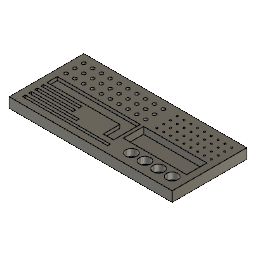
ToolingHolder1 v16 (Autodesk Fusion 360 design; units mm, degrees)
Autodesk Fusion 360 part; units mm, degrees
sketch "Sketch1" plane through (0, 0, 0) normal (0, 0, 1) x (1, 0, 0)
  line L0 (0, 0) -> (304.8, 0)
  line L1 (304.8, 0) -> (304.8, 139.7)
  line L2 (304.8, 139.7) -> (0, 139.7)
  line L3 (0, 139.7) -> (0, 0)
  dimension "d1" = 139.7
  dimension "d2" = 304.8
extrude "Extrude1" add sketch "Sketch1" along normal blind 19.05
sketch "Sketch2" plane through (0, 0, 19.05) normal (0, 0, 1) x (-1, 0, 0)
  line L0 (0, -139.7) -> (0, 0)
  line L1 (0, 0) -> (-304.8, 0)
  line L2 (-304.8, 0) -> (-304.8, -139.7)
  line L3 (-304.8, -139.7) -> (0, -139.7)
  line L4 (-304.8, -139.7) -> (0, -139.7)
  line L5 (-304.8, 0) -> (-304.8, -139.7)
  line L6 (0, 0) -> (-304.8, 0)
  line L7 (0, -139.7) -> (0, 0)
  line L8 (-12.7, -12.7) -> (-292.1, -12.7)
  line L9 (-292.1, -12.7) -> (-292.1, -127)
  line L10 (-292.1, -127) -> (-12.7, -127)
  line L11 (-12.7, -127) -> (-12.7, -12.7)
  circle A0 centre (-281.686, -23.114) radius 10.414
  circle A1 centre (-256.286, -23.114) radius 10.414
  line L12 (-12.7, -12.7) -> (-171.45, -12.7)
  line L13 (-171.45, -12.7) -> (-171.45, -17.78)
  line L14 (-171.45, -17.78) -> (-12.7, -17.78)
  line L15 (-12.7, -17.78) -> (-12.7, -12.7)
  line L16 (-12.7, -24.13) -> (-101.6, -24.13)
  line L17 (-101.6, -24.13) -> (-101.6, -29.21)
  line L18 (-101.6, -29.21) -> (-12.7, -29.21)
  line L19 (-12.7, -29.21) -> (-12.7, -24.13)
  line L20 (-12.7, -35.56) -> (-83.82, -35.56)
  line L21 (-83.82, -35.56) -> (-83.82, -40.64)
  line L22 (-83.82, -40.64) -> (-12.7, -40.64)
  line L23 (-12.7, -40.64) -> (-12.7, -35.56)
  line L24 (-12.7, -46.99) -> (-83.82, -46.99)
  line L25 (-83.82, -46.99) -> (-83.82, -52.07)
  line L26 (-83.82, -52.07) -> (-12.7, -52.07)
  line L27 (-12.7, -52.07) -> (-12.7, -46.99)
  circle A2 centre (-230.886, -23.114) radius 10.414
  circle A3 centre (-205.486, -23.114) radius 10.414
  line L28 (-12.7, -77.47) -> (-167.64, -77.47)
  line L29 (-167.64, -77.47) -> (-167.64, -27.615)
  line L30 (-167.64, -27.615) -> (-148.59, -27.615)
  line L31 (-148.59, -27.615) -> (-148.59, -58.42)
  line L32 (-148.59, -58.42) -> (-12.7, -58.42)
  circle A4 centre (-15.875, -123.825) radius 3.175
  circle A5 centre (-32.385, -123.825) radius 3.175
  circle A6 centre (-48.895, -123.825) radius 3.175
  circle A7 centre (-65.405, -123.825) radius 3.175
  circle A8 centre (-81.915, -123.825) radius 3.175
  circle A9 centre (-98.425, -123.825) radius 3.175
  circle A10 centre (-114.935, -123.825) radius 3.175
  circle A11 centre (-131.445, -123.825) radius 3.175
  circle A12 centre (-147.955, -123.825) radius 3.175
  circle A13 centre (-164.465, -123.825) radius 3.175
  circle A14 centre (-15.875, -107.315) radius 3.175
  circle A15 centre (-32.385, -107.315) radius 3.175
  circle A16 centre (-48.895, -107.315) radius 3.175
  circle A17 centre (-65.405, -107.315) radius 3.175
  circle A18 centre (-81.915, -107.315) radius 3.175
  circle A19 centre (-98.425, -107.315) radius 3.175
  circle A20 centre (-114.935, -107.315) radius 3.175
  circle A21 centre (-131.445, -107.315) radius 3.175
  circle A22 centre (-147.955, -107.315) radius 3.175
  circle A23 centre (-164.465, -107.315) radius 3.175
  circle A24 centre (-15.875, -90.805) radius 3.175
  circle A25 centre (-32.385, -90.805) radius 3.175
  circle A26 centre (-48.895, -90.805) radius 3.175
  circle A27 centre (-65.405, -90.805) radius 3.175
  circle A28 centre (-81.915, -90.805) radius 3.175
  circle A29 centre (-98.425, -90.805) radius 3.175
  circle A30 centre (-114.935, -90.805) radius 3.175
  circle A31 centre (-131.445, -90.805) radius 3.175
  circle A32 centre (-147.955, -90.805) radius 3.175
  circle A33 centre (-164.465, -90.805) radius 3.175
  circle A34 centre (-290.5125, -125.4125) radius 1.5875
  line L33 (-173.99, -77.47) -> (-292.1, -77.47)
  line L34 (-292.1, -77.47) -> (-292.1, -39.624)
  line L35 (-292.1, -39.624) -> (-173.99, -39.624)
  line L36 (-173.99, -39.624) -> (-173.99, -77.47)
  circle A35 centre (-277.8125, -125.4125) radius 1.5875
  circle A36 centre (-265.1125, -125.4125) radius 1.5875
  circle A37 centre (-252.4125, -125.4125) radius 1.5875
  circle A38 centre (-239.7125, -125.4125) radius 1.5875
  circle A39 centre (-227.0125, -125.4125) radius 1.5875
  circle A40 centre (-214.3125, -125.4125) radius 1.5875
  circle A41 centre (-201.6125, -125.4125) radius 1.5875
  circle A42 centre (-188.9125, -125.4125) radius 1.5875
  circle A43 centre (-290.5125, -112.7125) radius 1.5875
  circle A44 centre (-277.8125, -112.7125) radius 1.5875
  circle A45 centre (-265.1125, -112.7125) radius 1.5875
  circle A46 centre (-252.4125, -112.7125) radius 1.5875
  circle A47 centre (-239.7125, -112.7125) radius 1.5875
  circle A48 centre (-227.0125, -112.7125) radius 1.5875
  circle A49 centre (-214.3125, -112.7125) radius 1.5875
  circle A50 centre (-201.6125, -112.7125) radius 1.5875
  circle A51 centre (-188.9125, -112.7125) radius 1.5875
  circle A52 centre (-290.5125, -100.0125) radius 1.5875
  circle A53 centre (-277.8125, -100.0125) radius 1.5875
  circle A54 centre (-265.1125, -100.0125) radius 1.5875
  circle A55 centre (-252.4125, -100.0125) radius 1.5875
  circle A56 centre (-239.7125, -100.0125) radius 1.5875
  circle A57 centre (-227.0125, -100.0125) radius 1.5875
  circle A58 centre (-214.3125, -100.0125) radius 1.5875
  circle A59 centre (-201.6125, -100.0125) radius 1.5875
  circle A60 centre (-188.9125, -100.0125) radius 1.5875
  circle A61 centre (-290.5125, -87.3125) radius 1.5875
  circle A62 centre (-277.8125, -87.3125) radius 1.5875
  circle A63 centre (-265.1125, -87.3125) radius 1.5875
  circle A64 centre (-252.4125, -87.3125) radius 1.5875
  circle A65 centre (-239.7125, -87.3125) radius 1.5875
  circle A66 centre (-227.0125, -87.3125) radius 1.5875
  circle A67 centre (-214.3125, -87.3125) radius 1.5875
  circle A68 centre (-201.6125, -87.3125) radius 1.5875
  circle A69 centre (-188.9125, -87.3125) radius 1.5875
  dimension "d5" = 12.7
  dimension "d6" = 20.828
  dimension "d7" = 20.828
  dimension "d8" = 25.4
  dimension "d9" = 158.75
  dimension "d10" = 5.08
  dimension "d11" = 88.9
  dimension "d12" = 5.08
  dimension "d13" = 6.35
  dimension "d14" = 5.08
  dimension "d15" = 71.12
  dimension "d16" = 6.35
  dimension "d17" = 5.08
  dimension "d18" = 71.12
  dimension "d19" = 6.35
  dimension "d20" = 20.828
  dimension "d21" = 20.828
  dimension "d22" = 25.4
  dimension "d23" = 25.4
  dimension "d24" = 19.05
  dimension "d25" = 19.05
  dimension "d26" = 154.94
  dimension "d27" = 6.35
  dimension "d28" = 6.35
  dimension "d31" = -16.51
  dimension "d32" = 16.51
  dimension "d33" = 3.175
  dimension "d34" = 6.35
  dimension "d35" = 16.51
  dimension "d38" = 12.7
  dimension "d39" = 12.7
  measures "d6" diameter of A0
  measures "d7" diameter of A1
  measures "d11" distance of L0.end
  measures "d13" distance of L14 L16
  measures "d15" distance of L0.end
  measures "d16" distance of L18 L20
  measures "d18" distance of L0.end
  measures "d19" distance of L22 L24
  measures "d20" diameter of A2
  measures "d21" diameter of A3
  measures "d24" distance of L28 L32
  measures "d25" distance of L29 L31
  measures "d26" distance of L0.end
  measures "d27" distance of L26 L32
  measures "d28" diameter of A4
  measures "d33" diameter of A34
  measures "d34" distance of L29 L36
extrude "Extrude2" cut sketch "Sketch2" against normal blind 12.7 contours L8 L11 L12 L13 L14 L15 | A3 | A2 | A1 | A61 | A52 | A43 | A35 | A36 | A37 | A38 | A39 | A40 | A41 | A42 | A13 | A12 | A11 | A10 | A9 | A8 | A7 | A6 | A5 | A14 | A24 | L11 L16 L17 L18 L19 | L11 L20 L21 L22 L23 | A0 | L11 L24 L25 L26 L27 | L9 L33 L34 L35 L36 | A34 | A4 | A15 | A16 | A17 | A18 | A19 | A20 | A21 | A22 | A23 | A25 | A26 | A27 | A28 | A29 | A30 | A31 | A32 | A33 | A44 | A45 | A46 | A47 | A48 | A49 | A50 | A51 | A53 | A54 | A55 | A56 | A57 | A58 | A59 | A60 | A62 | A63 | A64 | A65 | A66 | A67 | A68 | A69
extrude "Extrude3" cut sketch "Sketch2" against normal blind 6.35 contours L11 L28 L29 L30 L31 L32
